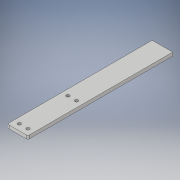
# Autodesk Inventor part: XZ chain support (flattened)
Saved by Autodesk Inventor 2018.2 (Build 222227000, 227)
## iProperties
Created: 2018-01-30
Part Number: XZ chain support (flattened)
Material: Generic
Document SubType Name: Modeling
Designer: torba
Density: 1 g/cm^3
Appearance: Default
Author: torba
Autodesk Inventor part; units mm, degrees
ref_plane "YZ Plane" through (0, 0, 0) normal (1, 0, 0) x (0, 1, 0)
ref_plane "XZ Plane" through (0, 0, 0) normal (0, 1, 0) x (-1, 0, 0)
ref_plane "XY Plane" through (0, 0, 0) normal (0, 0, 1) x (1, 0, 0)
sketch "Sketch1" plane through (0, 0, 0) normal (0, 1, 0) x (-1, 0, 0)
  line L0 (0, 0) -> (38.1, 0)
  line L1 (38.1, 0) -> (38.1, -268.6812)
  line L2 (38.1, -268.6812) -> (0, -268.6812)
  line L3 (0, -268.6812) -> (0, 0)
  circle A0 centre (11.05, -11.35) radius 3
  circle A1 centre (11.05, -101.35) radius 3
  circle A2 centre (27.05, -101.35) radius 3
  circle A3 centre (27.05, -11.35) radius 3
  arc A4 (3.175, 0) -> (0, -3.175) centre (3.175, -3.175) ccw
  line L4 (0, -3.175) -> (0, -110.9506)
  line L5 (38.1, -110.9506) -> (0, -110.9506) construction
  line L6 (38.1, -3.175) -> (38.1, -110.9506)
  arc A5 (38.1, -3.175) -> (34.925, 0) centre (34.925, -3.175) ccw
  line L7 (3.175, 0) -> (34.925, 0)
  point P0 (0, -48.7444)
  point P1 (19.05, 0)
  point P2 (19.05, 0)
  dimension "d0" = 38.1
  dimension "d1" = 268.6812
  dimension "d2" = 3.175
  dimension "d3" = 6
  dimension "d4" = 0
  dimension "d5" = 38.1
  dimension "d6" = 110.9506
  dimension "d7" = 110.9506
  dimension "d8" = 11.05
  dimension "d9" = 99.6006
  dimension "d10" = 11.05
  dimension "d11" = 9.6006
  dimension "d12" = 27.05
  dimension "d13" = 99.6006
  dimension "d14" = 27.05
  dimension "d15" = 9.6006
  dimension "d16" = 38.1
  dimension "d17" = 62.2062
  constraints: 16 end point, 6 centre point, 5 parallel, 4 equal radius, 4 point on circle, 4 tangent, 2 midpoint, 1 horizontal, 1 perpendicular, 1 vertical
  measures "d0" distance of L1.end L2.end
  measures "d1" distance of L0.end L1.end
  measures "d2" radius of A5
  measures "d3" diameter of A3
  measures "d4" distance between parallel lines of L6 L1
  measures "d5" distance between parallel lines of L6 L4
  measures "d6" distance between parallel lines of L5 L0
  measures "d7" distance between parallel lines of L5 L7
  measures "d8" distance from line of A3.centre L6
  measures "d9" distance from line of A3.centre L5
  measures "d10" distance from line of A2.centre L6
  measures "d11" distance from line of A2.centre L5
  measures "d12" distance from line of A0.centre L6
  measures "d13" distance from line of A0.centre L5
  measures "d14" distance from line of A1.centre L6
  measures "d15" distance from line of A1.centre L5
  measures "d16" distance from line of point (0, -48.744) L6
  measures "d17" distance from line of point (0, -48.744) L5
extrude "Extrusion1" add sketch "Sketch1" along normal blind 6.35
fillet "Fillet1" radius 3.175 2 edges at (0, 3.175, 0) (-38.1, 3.175, 0)
body "Solid1"
